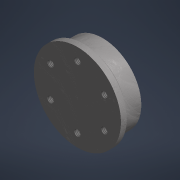
# Autodesk Inventor part: BridaTornillo2
Saved by Autodesk Inventor 2022 (Build 260153000, 153)
## iProperties
Created: 2021-09-22
Part Number: BridaTornillo2
Material: Steel, Mild, Welded
Document SubType Name: Modeling
Designer: Andres
Density: 7.85 g/cm^3
Appearance: Weld - Steel Mild
Mass: 118.114 g
Surface Area: 58.6184 cm^2
Volume: 15.0463 cm^3
Author: Andres
Autodesk Inventor part; units mm, degrees
ref_plane "YZ Plane" through (0, 0, 0) normal (1, 0, 0) x (0, 1, 0)
ref_plane "XZ Plane" through (0, 0, 0) normal (0, 1, 0) x (-1, 0, 0)
ref_plane "XY Plane" through (0, 0, 0) normal (0, 0, 1) x (1, 0, 0)
sketch "Sketch1" plane through (0, 0, 0) normal (0, 0, 1) x (1, 0, 0)
  point P0 (0, 0)
sketch "Sketch2" plane through (0, 0, 0) normal (0, 0, 1) x (1, 0, 0)
  circle A0 centre (0, 0) radius 8 projected
  circle A1 centre (0, 0) radius 20
  point P0 (0, 0)
  dimension "d26" = 40
  constraints: 1 centre point
  measures "d26" diameter of A1
extrude "Extrusion1" add sketch "Sketch2" against normal blind 10
sketch "Sketch3" plane through (0, 0, 0) normal (0, 0, 1) x (1, 0, 0)
  circle A0 centre (0, 0) radius 22.5
  dimension "d4" = 45
  constraints: 1 centre point, 1 coincident
  measures "d4" diameter of A0
extrude "Extrusion2" add sketch "Sketch3" along normal blind 3
ref_plane "Work Plane1" through (0.1016, -6, 78.7552) normal (0, -1, 0) x (1, 0, 0)
sketch "Sketch4" plane through (0.1016, -6, 78.7552) normal (0, -1, 0) x (1, 0, 0)
  arc A0 (1.5, -80.6705) -> (-1.5, -80.6705) centre (0, -80.6705) ccw projected
  line L0 (-1.5, -80.6705) -> (-1.5, -86.6705) projected
  line L1 (1.5, -86.6705) -> (1.5, -80.6705) projected
  arc A1 (-1.5, -86.6705) -> (1.5, -86.6705) centre (0, -86.6705) ccw projected
  line L2 (-1.5, -86.6705) -> (-1.5, -88.7552)
  line L3 (-1.5, -88.7552) -> (1.5, -88.7552)
  line L4 (1.5, -88.7552) -> (1.5, -86.6705)
  line L5 (-20.1016, -88.7552) -> (19.8984, -88.7552) projected
  line L6 (7.8984, -88.7552) -> (-8.1016, -88.7552) projected
  point P0 (-0.1016, -78.7552)
  point P1 (1.5, -80.6705)
  point P2 (-1.5, -80.6705)
  constraints: 6 end point, 1 collinear, 1 parallel, 1 perpendicular, 1 point on circle, 1 point on line
extrude "Extrusion3" cut sketch "Sketch4" along normal blind 3
sketch "Sketch5" plane through (0, 0, 0) normal (0, 0, -1) x (-1, 0, 0)
  circle A0 centre (0, 0) radius 22.5 projected
  circle A1 centre (0, 0) radius 20 projected
chamfer "Chamfer2" distance 2 angle 45 1 edges at (-20, 0, 0)
sketch "Sketch6" plane through (0, 0, 3) normal (0, 0, 1) x (1, 0, 0)
  circle A0 centre (0, 0) radius 16 construction
  point P0 (0, 16)
  dimension "d15" = 32
  constraints: 2 vertical alignment, 1 coincident, 2 other
hole "Hole1" at (0, 16, 3) direction (0, 0, -1) diameter 3.242 depth 11 tip angle 118 thread size "M4x0.7" class "6H" standard "ISO Metric profile"
pattern_circular "Circular Pattern1" count 6 over 360 about axis through (0, 0, 0) along (0, 0, 1) of "Hole1"
body "Solid1"
